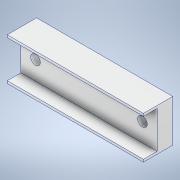
# Autodesk Inventor part: sensor
Saved by Autodesk Inventor 2022.1 (Build 261234000, 234)
## iProperties
Created: 2021-08-22
Part Number: sensor
Material: Aluminum 6061
Document SubType Name: Modeling
Designer: robst
Density: 2.7 g/cm^3
Appearance: Aluminum - Flat
Author: robst
Autodesk Inventor part; units mm, degrees
ref_plane "YZ Plane" through (0, 0, 0) normal (1, 0, 0) x (0, 1, 0)
ref_plane "XZ Plane" through (0, 0, 0) normal (0, 1, 0) x (-1, 0, 0)
ref_plane "XY Plane" through (0, 0, 0) normal (0, 0, 1) x (1, 0, 0)
sketch "Sketch1" plane through (0, 0, 0) normal (0, 0, 1) x (1, 0, 0)
  line L0 (-23.925, -7.425) -> (23.925, -7.425)
  line L1 (23.925, -7.425) -> (23.925, 7.425)
  line L2 (23.925, 7.425) -> (-23.925, 7.425)
  line L3 (-23.925, 7.425) -> (-23.925, -7.425)
  line L4 (-23.925, -7.425) -> (23.925, 7.425) construction
  line L5 (23.925, -7.425) -> (-23.925, 7.425) construction
  point P0 (0, 0)
  dimension "d0" = 47.85
  dimension "d1" = 14.85
  constraints: 12 end point, 2 midpoint, 2 parallel, 1 horizontal, 1 perpendicular
  measures "d0" distance of L0.start L0.end
  measures "d1" distance of L2.end L0.start
extrude "Extrusion1" add sketch "Sketch1" along normal blind 10.3
sketch "Sketch3" plane through (0, 0, 10.3) normal (0, 0, 1) x (1, 0, 0)
  line L0 (23.925, -7.425) -> (23.925, 7.425) projected
  line L1 (-23.925, 7.425) -> (-23.925, -7.425) projected
  line L2 (-23.925, -6.55) -> (23.925, -6.55)
  line L3 (23.925, -6.55) -> (23.925, 6.55)
  line L4 (23.925, 6.55) -> (-23.925, 6.55)
  line L5 (-23.925, 6.55) -> (-23.925, -6.55)
  line L6 (-23.925, -6.55) -> (23.925, 6.55) construction
  line L7 (23.925, -6.55) -> (-23.925, 6.55) construction
  point P0 (0, 0)
  dimension "d5" = 13.1
  constraints: 12 end point, 2 midpoint, 2 parallel, 1 collinear, 1 perpendicular
  measures "d5" distance between parallel lines of L2 L4
extrude "Extrusion2" cut sketch "Sketch3" against normal blind 4.8
sketch "Sketch4" plane through (0, 0, 5.5) normal (0, 0, 1) x (1, 0, 0)
  line L0 (-23.925, -6.55) -> (-23.925, 6.55) construction
  line L1 (-23.925, 0) -> (23.925, 0) construction
  line L2 (23.925, 6.55) -> (23.925, -6.55) construction
  point P0 (0, 0)
  point P1 (-18.8, 0)
  point P2 (18.8, 0)
  point P3 (0, 0)
  dimension "d8" = 18.8
  dimension "d9" = 18.8
  constraints: 3 midpoint, 2 end point, 2 point on line
  measures "d8" distance of point (-18.8, 0) point (0, 0)
  measures "d9" distance of point (18.8, 0) point (0, 0)
hole "Hole1" at (-18.8, 0, 5.5) at (18.8, 0, 5.5) direction (0, 0, -1) diameter 3.4 end through all clearance for "Flat Head Machine Screw" size "M3" standard "Ansi Metric M Profile"
equation "\"d0\" = sensorLength"
equation "\"d1\" = sensorWidth"
equation "\"d2\" = sensorDepth"
equation "\"d5\" = slotWidth"
equation "\"d6\" = slotDepth"
equation "\"d8\" = 0.5 * holeWidth"
equation "\"d9\" = 0.5 * holeWidth"
equation "\"sensorWidth\" = 14.85"
equation "\"sensorLength\" = 47.85"
equation "\"sensorDepth\" = 10.3"
equation "\"slotWidth\" = 13.1"
equation "\"slotDepth\" = 4.8"
equation "\"holeWidth\" = 37.6"
equation "\"holeDiameter\" = 3.4"
body "Solid1"
